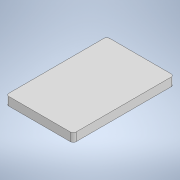
# Autodesk Inventor part: wheel_part
Saved by Autodesk Inventor 2022 (Build 260153000, 153)
## iProperties
Created: 2022-08-04
Part Number: wheel_part
Material: Generic
Document SubType Name: Modeling
Designer: Alok
Density: 1 g/cm^3
Appearance: Default
Author: Alok
Autodesk Inventor part; units mm, degrees
ref_plane "YZ Plane" through (0, 0, 0) normal (1, 0, 0) x (0, 1, 0)
ref_plane "XZ Plane" through (0, 0, 0) normal (0, 1, 0) x (-1, 0, 0)
ref_plane "XY Plane" through (0, 0, 0) normal (0, 0, 1) x (1, 0, 0)
sketch "Sketch1" plane through (0, 0, 0) normal (0, 1, 0) x (-1, 0, 0)
  line L0 (60, 90) -> (-60, 90)
  line L1 (-60, 90) -> (-60, -90)
  line L2 (-60, -90) -> (60, -90)
  line L3 (60, -90) -> (60, 90)
  line L4 (60, 90) -> (-60, -90) construction
  line L5 (-60, 90) -> (60, -90) construction
  point P0 (0, 0)
  dimension "d0" = 120
  dimension "d1" = 180
  constraints: 12 end point, 2 midpoint, 2 parallel, 1 horizontal, 1 perpendicular
  measures "d0" distance of L2.end L1.end
  measures "d1" distance of L1.end L0.end
extrude "Extrusion1" add sketch "Sketch1" along normal blind 15
fillet "Face Fillet1" radius 5 1 edges at (60, 7.5, 90)
fillet "Face Fillet2" radius 5 1 edges at (60, 7.5, -90)
fillet "Face Fillet3" radius 5 1 edges at (-60, 7.5, 90)
fillet "Face Fillet4" radius 5 1 edges at (-60, 7.5, -90)
body "Solid1"
